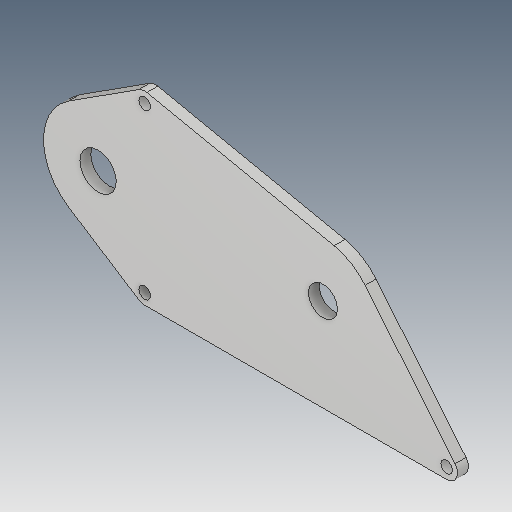
# Autodesk Inventor part: 支え
Saved by Autodesk Inventor 2019.4 (Build 234330000, 330)
## iProperties
Created: 2019-06-12
Part Number: 支え
Material: アルミニウム 2014-T4
Document SubType Name: Modeling
Designer: AzLIer
Density: 2.8 g/cm^3
Appearance: サテン
Mass: 33.3873 g
Surface Area: 90.2364 cm^2
Volume: 11.924 cm^3
Author: AzLIer
Autodesk Inventor part; units mm, degrees
(part 1 of 3)
ref_plane "YZ Plane" through (0, 0, 0) normal (1, 0, 0) x (0, 1, 0)
ref_plane "XZ Plane" through (0, 0, 0) normal (0, 1, 0) x (-1, 0, 0)
ref_plane "XY Plane" through (0, 0, 0) normal (0, 0, 1) x (1, 0, 0)
sketch "スケッチ1" plane through (0, 0, 0) normal (0, 0, 1) x (1, 0, 0)
  circle A0 centre (-1.8122, 42.5) radius 4 construction
  circle A1 centre (60, 42.5) radius 4
  circle A2 centre (0, 0) radius 1.6 construction
  circle A3 centre (120, 0) radius 1.6 construction
  circle A4 centre (-1.8122, 42.5) radius 6 construction
  circle A5 centre (120, 0) radius 1.6 construction
  circle A6 centre (0, 0) radius 1.6 construction
  line L0 (-60, -7.5) -> (5, -7.5) construction
  line L1 (5, -7.5) -> (5, 2.5) construction
  line L2 (5, 2.5) -> (115, 2.5) construction
  line L3 (115, 2.5) -> (115, -7.5) construction
  line L4 (115, -7.5) -> (180, -7.5) construction
  circle A7 centre (60, 42.5) radius 9.5 construction
  circle A8 centre (-1.8122, 42.5) radius 5
  arc A9 (-27.1122, 50.5) -> (-27.1122, 47.5) centre (-27.1122, 49) ccw construction
  line L5 (-27.1122, 50.5) -> (-24.1122, 50.5) construction
  arc A10 (-24.1122, 47.5) -> (-24.1122, 50.5) centre (-24.1122, 49) ccw construction
  line L6 (-24.1122, 47.5) -> (-24.1122, 37.5) construction
  arc A11 (-24.1122, 34.5) -> (-24.1122, 37.5) centre (-24.1122, 36) ccw construction
  line L7 (-24.1122, 34.5) -> (-27.1122, 34.5) construction
  arc A12 (-27.1122, 37.5) -> (-27.1122, 34.5) centre (-27.1122, 36) ccw construction
  line L8 (-27.1122, 37.5) -> (-27.1122, 47.5) construction
  circle A13 centre (-30.1122, 42.5) radius 1.6 construction
  arc A14 (-43.1122, 50.5) -> (-43.1122, 47.5) centre (-43.1122, 49) ccw construction
  line L9 (-43.1122, 50.5) -> (-40.1122, 50.5) construction
  arc A15 (-40.1122, 47.5) -> (-40.1122, 50.5) centre (-40.1122, 49) ccw construction
  line L10 (-40.1122, 47.5) -> (-40.1122, 37.5) construction
  arc A16 (-40.1122, 34.5) -> (-40.1122, 37.5) centre (-40.1122, 36) ccw construction
  line L11 (-40.1122, 34.5) -> (-43.1122, 34.5) construction
  arc A17 (-43.1122, 37.5) -> (-43.1122, 34.5) centre (-43.1122, 36) ccw construction
  line L12 (-43.1122, 37.5) -> (-43.1122, 47.5) construction
  circle A18 centre (-46.1122, 42.5) radius 1.6 construction
  arc A19 (32.7108, 25.7878) -> (79.8762, 17.4214) centre (60, 42.5) ccw construction
  arc A20 (33.6707, 28.6881) -> (32.7108, 25.7878) centre (34.4163, 26.8323) ccw construction
  line L13 (33.6707, 28.6881) -> (46.0418, 33.6587) construction
  arc A21 (48.3419, 33.0614) -> (46.0418, 33.6587) centre (46.7874, 31.8029) ccw construction
  arc A22 (48.3419, 33.0614) -> (71.3533, 32.6969) centre (60, 42.5) ccw construction
  arc A23 (74.6806, 32.2331) -> (71.3533, 32.6969) centre (72.8671, 31.3898) ccw construction
  line L14 (74.6806, 32.2331) -> (80.4475, 19.8322) construction
  arc A24 (79.8762, 17.4214) -> (80.4475, 19.8322) centre (78.634, 18.9888) ccw construction
  arc A25 (45.2156, 45.0341) -> (45.0523, 41.2488) centre (60, 42.5) ccw construction
  arc A26 (43.8049, 39.2261) -> (45.0523, 41.2488) centre (43.0592, 41.0819) ccw construction
  line L15 (43.8049, 39.2261) -> (31.4338, 34.2556) construction
  arc A27 (28.734, 35.6855) -> (31.4338, 34.2556) centre (30.6881, 36.1114) ccw construction
  arc A28 (28.3012, 38.1199) -> (28.734, 35.6855) centre (60, 42.5) ccw construction
  arc A29 (28.2895, 38.5625) -> (28.3012, 38.1199) centre (30.2824, 38.3937) ccw construction
  line L16 (28.2895, 38.5625) -> (29.8074, 56.4773) construction
  arc A30 (33.182, 57.7544) -> (29.8074, 56.4773) centre (31.8002, 56.3085) ccw construction
  line L17 (33.182, 57.7544) -> (44.6261, 46.8179) construction
  arc A31 (45.2156, 45.0341) -> (44.6261, 46.8179) centre (43.2444, 45.372) ccw construction
  arc A32 (37.2786, 112.9254) -> (13.7146, 100.2379) centre (60, 42.5) ccw construction
  arc A33 (39.8605, 111.3796) -> (37.2786, 112.9254) centre (37.8927, 111.022) ccw construction
  line L18 (39.8605, 111.3796) -> (47.3934, 69.926) construction
  arc A34 (44.0438, 68.1225) -> (47.3934, 69.926) centre (45.4256, 69.5684) ccw construction
  line L19 (44.0438, 68.1225) -> (13.5837, 97.2315) construction
  arc A35 (13.7146, 100.2379) -> (13.5837, 97.2315) centre (14.9655, 98.6774) ccw construction
  circle A36 centre (60, 42.5) radius 4 construction
  circle A37 centre (24.575, 76.3537) radius 1.2295 construction
  circle A38 centre (51.2393, 90.7105) radius 1.2295 construction
  circle A39 centre (53.9211, 75.9522) radius 1.2295 construction
  circle A40 centre (35.4194, 65.9903) radius 1.2295 construction
  arc A41 (53.4682, 120.3931) -> (51.2825, 122.0236) centre (51.5004, 120.0355) ccw construction
  arc A42 (51.2825, 122.0236) -> (-1.5901, 93.5555) centre (60, 42.5) ccw construction
  arc A43 (-1.5901, 93.5555) -> (-1.4321, 90.8332) centre (-0.0503, 92.2791) ccw construction
  line L20 (-1.4321, 90.8332) -> (23.8669, 66.6564) construction
  arc A44 (24.4709, 64.9726) -> (23.8669, 66.6564) centre (22.4851, 65.2105) ccw construction
  line L21 (24.4709, 64.9726) -> (22.8037, 51.0517) construction
  arc A45 (20.4778, 49.3186) -> (22.8037, 51.0517) centre (20.8179, 51.2895) ccw construction
  line L22 (20.4778, 49.3186) -> (10.913, 50.9688) construction
  line L23 (10.913, 50.9688) -> (10.8526, 50.6108) construction
  line L24 (10.8526, 50.6108) -> (10.7948, 50.2524) construction
  line L25 (10.7948, 50.2524) -> (10.7396, 49.8936) construction
  line L26 (10.7396, 49.8936) -> (10.687, 49.5343) construction
  line L27 (10.687, 49.5343) -> (10.6371, 49.1747) construction
  line L28 (10.6371, 49.1747) -> (10.5897, 48.8148) construction
  line L29 (10.5897, 48.8148) -> (10.545, 48.4545) construction
  line L30 (10.545, 48.4545) -> (10.5029, 48.0939) construction
  line L31 (10.5029, 48.0939) -> (10.4635, 47.733) construction
  line L32 (10.4635, 47.733) -> (10.4266, 47.3718) construction
  line L33 (10.4266, 47.3718) -> (10.7788, 47.1061) construction
  line L34 (10.7788, 47.1061) -> (11.1328, 46.8484) construction
  line L35 (11.1328, 46.8484) -> (11.4885, 46.5989) construction
  line L36 (11.4885, 46.5989) -> (11.8459, 46.3577) construction
  line L37 (11.8459, 46.3577) -> (12.2048, 46.1249) construction
  line L38 (12.2048, 46.1249) -> (12.5653, 45.9007) construction
  line L39 (12.5653, 45.9007) -> (12.9271, 45.6853) construction
  line L40 (12.9271, 45.6853) -> (13.2903, 45.4788) construction
  line L41 (13.2903, 45.4788) -> (13.6547, 45.2815) construction
  line L42 (13.6547, 45.2815) -> (14.0204, 45.0936) construction
  line L43 (14.0204, 45.0936) -> (14.3872, 44.9154) construction
  line L44 (14.3872, 44.9154) -> (14.755, 44.7473) construction
  line L45 (14.755, 44.7473) -> (15.1238, 44.5897) construction
  line L46 (15.1238, 44.5897) -> (15.4935, 44.4431) construction
  line L47 (15.4935, 44.4431) -> (15.8641, 44.3081) construction
  line L48 (15.8641, 44.3081) -> (16.2354, 44.1857) construction
  line L49 (16.2354, 44.1857) -> (16.6076, 44.077) construction
  line L50 (16.6076, 44.077) -> (16.9805, 43.9839) construction
  line L51 (16.9805, 43.9839) -> (17.3541, 43.9096) construction
  line L52 (17.3541, 43.9096) -> (17.7287, 43.863) construction
  line L53 (17.7287, 43.863) -> (18.0074, 43.843) construction
  line L54 (18.0074, 43.843) -> (18.2771, 43.8116) construction
  line L55 (18.2771, 43.8116) -> (18.5376, 43.771) construction
  line L56 (18.5376, 43.771) -> (18.7888, 43.724) construction
  line L57 (18.7888, 43.724) -> (19.0304, 43.665) construction
  line L58 (19.0304, 43.665) -> (19.2623, 43.5939) construction
  line L59 (19.2623, 43.5939) -> (19.4841, 43.5104) construction
  line L60 (19.4841, 43.5104) -> (19.6958, 43.4209) construction
  line L61 (19.6958, 43.4209) -> (19.897, 43.319) construction
  line L62 (19.897, 43.319) -> (20.0874, 43.2026) construction
  line L63 (20.0874, 43.2026) -> (20.2667, 43.0791) construction
  line L64 (20.2667, 43.0791) -> (20.4346, 42.9419) construction
  line L65 (20.4346, 42.9419) -> (20.5905, 42.7916) construction
  line L66 (20.5905, 42.7916) -> (20.7341, 42.6315) construction
  line L67 (20.7341, 42.6315) -> (20.8645, 42.4541) construction
  line L68 (20.8645, 42.4541) -> (20.9809, 42.2667) construction
  line L69 (20.9809, 42.2667) -> (21.0822, 42.0577) construction
  line L70 (21.0822, 42.0577) -> (21.1667, 41.8325) construction
  line L71 (21.1667, 41.8325) -> (21.2319, 41.5673) construction
  line L72 (21.2319, 41.5673) -> (21.2711, 41.2223) construction
  line L73 (21.2711, 41.2223) -> (21.2729, 41.1669) construction
  line L74 (21.2729, 41.1669) -> (21.2749, 41.1115) construction
  line L75 (21.2749, 41.1115) -> (21.2769, 41.0561) construction
  line L76 (21.2769, 41.0561) -> (21.279, 41.0007) construction
  line L77 (21.279, 41.0007) -> (21.2812, 40.9454) construction
  line L78 (21.2812, 40.9454) -> (21.2835, 40.89) construction
  line L79 (21.2835, 40.89) -> (21.2858, 40.8346) construction
  line L80 (21.2858, 40.8346) -> (21.2882, 40.7793) construction
  line L81 (21.2882, 40.7793) -> (21.2907, 40.7239) construction
  line L82 (21.2907, 40.7239) -> (21.2933, 40.6685) construction
  line L83 (21.2933, 40.6685) -> (21.2819, 40.3215) construction
  line L84 (21.2819, 40.3215) -> (21.2382, 40.0519) construction
  line L85 (21.2382, 40.0519) -> (21.1721, 39.8207) construction
  line L86 (21.1721, 39.8207) -> (21.0878, 39.6042) construction
  line L87 (21.0878, 39.6042) -> (20.9868, 39.4081) construction
  line L88 (20.9868, 39.4081) -> (20.871, 39.2208) construction
  line L89 (20.871, 39.2208) -> (20.7408, 39.0497) construction
  line L90 (20.7408, 39.0497) -> (20.5974, 38.8874) construction
  line L91 (20.5974, 38.8874) -> (20.4411, 38.7371) construction
  line L92 (20.4411, 38.7371) -> (20.2722, 38.5997) construction
  line L93 (20.2722, 38.5997) -> (20.0917, 38.4684) construction
  line L94 (20.0917, 38.4684) -> (19.8994, 38.3507) construction
  line L95 (19.8994, 38.3507) -> (19.6955, 38.2445) construction
  line L96 (19.6955, 38.2445) -> (19.4811, 38.1435) construction
  line L97 (19.4811, 38.1435) -> (19.2557, 38.054) construction
  line L98 (19.2557, 38.054) -> (19.0196, 37.9758) construction
  line L99 (19.0196, 37.9758) -> (18.7729, 37.9089) construction
  line L100 (18.7729, 37.9089) -> (18.5165, 37.8475) construction
  line L101 (18.5165, 37.8475) -> (18.2503, 37.7946) construction
  line L102 (18.2503, 37.7946) -> (17.9741, 37.7523) construction
  line L103 (17.9741, 37.7523) -> (17.6044, 37.6758) construction
  line L104 (17.6044, 37.6758) -> (17.2379, 37.5718) construction
  line L105 (17.2379, 37.5718) -> (16.8737, 37.4491) construction
  line L106 (16.8737, 37.4491) -> (16.5115, 37.3109) construction
  line L107 (16.5115, 37.3109) -> (16.1511, 37.1591) construction
  line L108 (16.1511, 37.1591) -> (15.7926, 36.9949) construction
  line L109 (15.7926, 36.9949) -> (15.4358, 36.8191) construction
  line L110 (15.4358, 36.8191) -> (15.0808, 36.6324) construction
  line L111 (15.0808, 36.6324) -> (14.7277, 36.4354) construction
  line L112 (14.7277, 36.4354) -> (14.3764, 36.2284) construction
  line L113 (14.3764, 36.2284) -> (14.0269, 36.0118) construction
  line L114 (14.0269, 36.0118) -> (13.6795, 35.7859) construction
  line L115 (13.6795, 35.7859) -> (13.334, 35.5509) construction
  line L116 (13.334, 35.5509) -> (12.9906, 35.3072) construction
  line L117 (12.9906, 35.3072) -> (12.6493, 35.0548) construction
  line L118 (12.6493, 35.0548) -> (12.3102, 34.794) construction
  line L119 (12.3102, 34.794) -> (11.9733, 34.5249) construction
  line L120 (11.9733, 34.5249) -> (11.6388, 34.2477) construction
  line L121 (11.6388, 34.2477) -> (11.3066, 33.9624) construction
  line L122 (11.3066, 33.9624) -> (10.9768, 33.6693) construction
  line L123 (10.9768, 33.6693) -> (11.0425, 33.3123) construction
  line L124 (11.0425, 33.3123) -> (11.1108, 32.9557) construction
  line L125 (11.1108, 32.9557) -> (11.1816, 32.5996) construction
  line L126 (11.1816, 32.5996) -> (11.2551, 32.2441) construction
  line L127 (11.2551, 32.2441) -> (11.3311, 31.8891) construction
  line L128 (11.3311, 31.8891) -> (11.4097, 31.5347) construction
  line L129 (11.4097, 31.5347) -> (11.491, 31.1808) construction
  line L130 (11.491, 31.1808) -> (11.5747, 30.8275) construction
  line L131 (11.5747, 30.8275) -> (11.6611, 30.4749) construction
  line L132 (11.6611, 30.4749) -> (11.75, 30.1229) construction
  line L133 (11.75, 30.1229) -> (12.1718, 29.9937) construction
  line L134 (12.1718, 29.9937) -> (12.5926, 29.8726) construction
  line L135 (12.5926, 29.8726) -> (13.0122, 29.7598) construction
  line L136 (13.0122, 29.7598) -> (13.4305, 29.6554) construction
  line L137 (13.4305, 29.6554) -> (13.8474, 29.5594) construction
  line L138 (13.8474, 29.5594) -> (14.2628, 29.472) construction
  line L139 (14.2628, 29.472) -> (14.6765, 29.3933) construction
  line L140 (14.6765, 29.3933) -> (15.0884, 29.3235) construction
  line L141 (15.0884, 29.3235) -> (15.4984, 29.2627) construction
  line L142 (15.4984, 29.2627) -> (15.9062, 29.2112) construction
  line L143 (15.9062, 29.2112) -> (16.3118, 29.1692) construction
  line L144 (16.3118, 29.1692) -> (16.715, 29.1371) construction
  line L145 (16.715, 29.1371) -> (17.1154, 29.1151) construction
  line L146 (17.1154, 29.1151) -> (17.513, 29.1038) construction
  line L147 (17.513, 29.1038) -> (17.9074, 29.1037) construction
  line L148 (17.9074, 29.1037) -> (18.2982, 29.1157) construction
  line L149 (18.2982, 29.1157) -> (18.6851, 29.1409) construction
  line L150 (18.6851, 29.1409) -> (19.0673, 29.1809) construction
  line L151 (19.0673, 29.1809) -> (19.4439, 29.2388) construction
  line L152 (19.4439, 29.2388) -> (19.8118, 29.3232) construction
  line L153 (19.8118, 29.3232) -> (20.0806, 29.3997) construction
  line L154 (20.0806, 29.3997) -> (20.3447, 29.4625) construction
  line L155 (20.3447, 29.4625) -> (20.6033, 29.5133) construction
  line L156 (20.6033, 29.5133) -> (20.8555, 29.5551) construction
  line L157 (20.8555, 29.5551) -> (21.1027, 29.5823) construction
  line L158 (21.1027, 29.5823) -> (21.3449, 29.5948) construction
  line L159 (21.3449, 29.5948) -> (21.5819, 29.5922) construction
  line L160 (21.5819, 29.5922) -> (21.8115, 29.5805) construction
  line L161 (21.8115, 29.5805) -> (22.0354, 29.5535) construction
  line L162 (22.0354, 29.5535) -> (22.2541, 29.5093) construction
  line L163 (22.2541, 29.5093) -> (22.4649, 29.4546) construction
  line L164 (22.4649, 29.4546) -> (22.6695, 29.3831) construction
  line L165 (22.6695, 29.3831) -> (22.8675, 29.2952) construction
  line L166 (22.8675, 29.2952) -> (23.0571, 29.1938) construction
  line L167 (23.0571, 29.1938) -> (23.2403, 29.0717) construction
  line L168 (23.2403, 29.0717) -> (23.4138, 28.9355) construction
  line L169 (23.4138, 28.9355) -> (23.5805, 28.7737) construction
  line L170 (23.5805, 28.7737) -> (23.737, 28.591) construction
  line L171 (23.737, 28.591) -> (23.8889, 28.3641) construction
  line L172 (23.8889, 28.3641) -> (24.0437, 28.0533) construction
  line L173 (24.0437, 28.0533) -> (24.0644, 28.0018) construction
  line L174 (24.0644, 28.0018) -> (24.0852, 27.9505) construction
  line L175 (24.0852, 27.9505) -> (24.106, 27.8991) construction
  line L176 (24.106, 27.8991) -> (24.127, 27.8478) construction
  line L177 (24.127, 27.8478) -> (24.1479, 27.7965) construction
  line L178 (24.1479, 27.7965) -> (24.169, 27.7453) construction
  line L179 (24.169, 27.7453) -> (24.1901, 27.694) construction
  line L180 (24.1901, 27.694) -> (24.2114, 27.6428) construction
  line L181 (24.2114, 27.6428) -> (24.2326, 27.5917) construction
  line L182 (24.2326, 27.5917) -> (24.254, 27.5405) construction
  line L183 (24.254, 27.5405) -> (24.362, 27.2105) construction
  line L184 (24.362, 27.2105) -> (24.4132, 26.9422) construction
  line L185 (24.4132, 26.9422) -> (24.4301, 26.7023) construction
  line L186 (24.4301, 26.7023) -> (24.4249, 26.4701) construction
  line L187 (24.4249, 26.4701) -> (24.397, 26.2513) construction
  line L188 (24.397, 26.2513) -> (24.3523, 26.0357) construction
  line L189 (24.3523, 26.0357) -> (24.2885, 25.8303) construction
  line L190 (24.2885, 25.8303) -> (24.2092, 25.6287) construction
  line L191 (24.2092, 25.6287) -> (24.1137, 25.4341) construction
  line L192 (24.1137, 25.4341) -> (24.0021, 25.2472) construction
  line L193 (24.0021, 25.2472) -> (23.8774, 25.0621) construction
  line L194 (23.8774, 25.0621) -> (23.7369, 24.8857) construction
  line L195 (23.7369, 24.8857) -> (23.5816, 24.7162) construction
  line L196 (23.5816, 24.7162) -> (23.4147, 24.5479) construction
  line L197 (23.4147, 24.5479) -> (23.2335, 24.3868) construction
  line L198 (23.2335, 24.3868) -> (23.0384, 24.2326) construction
  line L199 (23.0384, 24.2326) -> (22.8295, 24.0853) construction
  line L200 (22.8295, 24.0853) -> (22.6096, 23.9399) construction
  line L201 (22.6096, 23.9399) -> (22.3774, 23.7991) construction
  line L202 (22.3774, 23.7991) -> (22.1324, 23.6649) construction
  line L203 (22.1324, 23.6649) -> (21.8111, 23.4666) construction
  line L204 (21.8111, 23.4666) -> (21.5024, 23.2435) construction
  line L205 (21.5024, 23.2435) -> (21.2021, 23.0036) construction
  line L206 (21.2021, 23.0036) -> (20.9089, 22.7499) construction
  line L207 (20.9089, 22.7499) -> (20.6222, 22.484) construction
  line L208 (20.6222, 22.484) -> (20.3415, 22.207) construction
  line L209 (20.3415, 22.207) -> (20.0663, 21.9198) construction
  line L210 (20.0663, 21.9198) -> (19.7966, 21.623) construction
  line L211 (19.7966, 21.623) -> (19.5321, 21.3171) construction
  line L212 (19.5321, 21.3171) -> (19.2728, 21.0024) construction
  line L213 (19.2728, 21.0024) -> (19.0186, 20.6793) construction
  line L214 (19.0186, 20.6793) -> (18.7693, 20.3482) construction
  line L215 (18.7693, 20.3482) -> (18.5251, 20.0093) construction
  line L216 (18.5251, 20.0093) -> (18.2857, 19.6628) construction
  line L217 (18.2857, 19.6628) -> (18.0513, 19.3089) construction
  line L218 (18.0513, 19.3089) -> (17.8219, 18.9478) construction
  line L219 (17.8219, 18.9478) -> (17.5973, 18.5798) construction
  line L220 (17.5973, 18.5798) -> (17.3778, 18.2048) construction
  line L221 (17.3778, 18.2048) -> (17.1632, 17.8232) construction
  line L222 (17.1632, 17.8232) -> (16.9535, 17.435) construction
  line L223 (16.9535, 17.435) -> (17.1374, 17.1219) construction
  line L224 (17.1374, 17.1219) -> (17.3235, 16.8102) construction
  line L225 (17.3235, 16.8102) -> (17.5119, 16.4998) construction
  line L226 (17.5119, 16.4998) -> (17.7025, 16.1908) construction
  line L227 (17.7025, 16.1908) -> (17.8954, 15.8833) construction
  line L228 (17.8954, 15.8833) -> (18.0905, 15.5771) construction
  line L229 (18.0905, 15.5771) -> (18.2878, 15.2724) construction
  line L230 (18.2878, 15.2724) -> (18.4874, 14.9691) construction
  line L231 (18.4874, 14.9691) -> (18.6891, 14.6672) construction
  line L232 (18.6891, 14.6672) -> (18.8931, 14.3669) construction
  line L233 (18.8931, 14.3669) -> (19.3337, 14.3897) construction
  line L234 (19.3337, 14.3897) -> (19.7705, 14.4199) construction
  line L235 (19.7705, 14.4199) -> (20.2033, 14.4574) construction
  line L236 (20.2033, 14.4574) -> (20.6321, 14.5023) construction
  line L237 (20.6321, 14.5023) -> (21.0567, 14.5547) construction
  line L238 (21.0567, 14.5547) -> (21.4769, 14.6146) construction
  line L239 (21.4769, 14.6146) -> (21.8926, 14.6822) construction
  line L240 (21.8926, 14.6822) -> (22.3036, 14.7575) construction
  line L241 (22.3036, 14.7575) -> (22.7096, 14.8406) construction
  line L242 (22.7096, 14.8406) -> (23.1105, 14.9317) construction
  line L243 (23.1105, 14.9317) -> (23.5059, 15.031) construction
  line L244 (23.5059, 15.031) -> (23.8958, 15.1386) construction
  line L245 (23.8958, 15.1386) -> (24.2796, 15.2549) construction
  line L246 (24.2796, 15.2549) -> (24.657, 15.3803) construction
  line L247 (24.657, 15.3803) -> (25.0277, 15.5151) construction
  line L248 (25.0277, 15.5151) -> (25.3908, 15.66) construction
  line L249 (25.3908, 15.66) -> (25.7458, 15.816) construction
  line L250 (25.7458, 15.816) -> (26.0913, 15.9843) construction
  line L251 (26.0913, 15.9843) -> (26.4253, 16.1676) construction
  line L252 (26.4253, 16.1676) -> (26.7422, 16.3727) construction
  line L253 (26.7422, 16.3727) -> (26.9686, 16.5365) construction
  line L254 (26.9686, 16.5365) -> (27.1953, 16.6858) construction
  line L255 (27.1953, 16.6858) -> (27.421, 16.8221) construction
  line L256 (27.421, 16.8221) -> (27.6436, 16.9476) construction
  line L257 (27.6436, 16.9476) -> (27.8666, 17.0577) construction
  line L258 (27.8666, 17.0577) -> (28.0899, 17.1523) construction
  line L259 (28.0899, 17.1523) -> (28.3135, 17.2309) construction
  line L260 (28.3135, 17.2309) -> (28.5333, 17.2984) construction
  line L261 (28.5333, 17.2984) -> (28.7529, 17.3496) construction
  line L262 (28.7529, 17.3496) -> (28.9735, 17.3829) construction
  line L263 (28.9735, 17.3829) -> (29.1903, 17.4036) construction
  line L264 (29.1903, 17.4036) -> (29.4071, 17.4064) construction
  line L265 (29.4071, 17.4064) -> (29.6231, 17.3915) construction
  line L266 (29.6231, 17.3915) -> (29.836, 17.3611) construction
  line L267 (29.836, 17.3611) -> (30.05, 17.309) construction
  line L268 (30.05, 17.309) -> (30.2596, 17.2403) construction
  line L269 (30.2596, 17.2403) -> (30.4716, 17.1453) construction
  line L270 (30.4716, 17.1453) -> (30.6811, 17.0271) construction
  line L271 (30.6811, 17.0271) -> (30.9014, 16.8658) construction
  line L272 (30.9014, 16.8658) -> (31.1532, 16.6267) construction
  line L273 (31.1532, 16.6267) -> (31.1903, 16.5855) construction
  line L274 (31.1903, 16.5855) -> (31.2274, 16.5443) construction
  line L275 (31.2274, 16.5443) -> (31.2645, 16.5032) construction
  line L276 (31.2645, 16.5032) -> (31.3017, 16.4621) construction
  line L277 (31.3017, 16.4621) -> (31.339, 16.4211) construction
  line L278 (31.339, 16.4211) -> (31.3763, 16.3802) construction
  line L279 (31.3763, 16.3802) -> (31.4137, 16.3392) construction
  line L280 (31.4137, 16.3392) -> (31.4511, 16.2984) construction
  line L281 (31.4511, 16.2984) -> (31.4886, 16.2576) construction
  line L282 (31.4886, 16.2576) -> (31.5262, 16.2168) construction
  line L283 (31.5262, 16.2168) -> (31.7405, 15.9436) construction
  line L284 (31.7405, 15.9436) -> (31.8804, 15.7091) construction
  line L285 (31.8804, 15.7091) -> (31.9783, 15.4894) construction
  line L286 (31.9783, 15.4894) -> (32.0529, 15.2694) construction
  line L287 (32.0529, 15.2694) -> (32.1016, 15.0543) construction
  line L288 (32.1016, 15.0543) -> (32.1333, 14.8364) construction
  line L289 (32.1333, 14.8364) -> (32.1435, 14.6216) construction
  line L290 (32.1435, 14.6216) -> (32.138, 14.405) construction
  line L291 (32.138, 14.405) -> (32.1148, 14.1895) construction
  line L292 (32.1148, 14.1895) -> (32.0738, 13.9756) construction
  line L293 (32.0738, 13.9756) -> (32.0199, 13.7591) construction
  line L294 (32.0199, 13.7591) -> (31.9482, 13.5453) construction
  line L295 (31.9482, 13.5453) -> (31.8604, 13.3329) construction
  line L296 (31.8604, 13.3329) -> (31.761, 13.1177) construction
  line L297 (31.761, 13.1177) -> (31.6459, 12.9043) construction
  line L298 (31.6459, 12.9043) -> (31.5153, 12.6926) construction
  line L299 (31.5153, 12.6926) -> (31.3694, 12.4827) construction
  line L300 (31.3694, 12.4827) -> (31.2124, 12.2709) construction
  line L301 (31.2124, 12.2709) -> (31.0424, 12.0593) construction
  line L302 (31.0424, 12.0593) -> (30.8581, 11.8493) construction
  line L303 (30.8581, 11.8493) -> (30.624, 11.5531) construction
  line L304 (30.624, 11.5531) -> (30.4102, 11.2378) construction
  line L305 (30.4102, 11.2378) -> (30.21, 10.9097) construction
  line L306 (30.21, 10.9097) -> (30.0214, 10.571) construction
  line L307 (30.0214, 10.571) -> (29.8429, 10.2231) construction
  line L308 (29.8429, 10.2231) -> (29.6738, 9.8668) construction
  line L309 (29.6738, 9.8668) -> (29.5134, 9.5029) construction
  line L310 (29.5134, 9.5029) -> (29.3615, 9.1317) construction
  line L311 (29.3615, 9.1317) -> (29.2176, 8.7537) construction
  line L312 (29.2176, 8.7537) -> (29.0816, 8.3693) construction
  line L313 (29.0816, 8.3693) -> (28.9532, 7.9788) construction
  line L314 (28.9532, 7.9788) -> (28.8322, 7.5824) construction
  line L315 (28.8322, 7.5824) -> (28.7186, 7.1804) construction
  line L316 (28.7186, 7.1804) -> (28.6122, 6.7729) construction
  line L317 (28.6122, 6.7729) -> (28.513, 6.3602) construction
  line L318 (28.513, 6.3602) -> (28.4208, 5.9424) construction
  line L319 (28.4208, 5.9424) -> (28.3357, 5.5198) construction
  line L320 (28.3357, 5.5198) -> (28.2576, 5.0923) construction
  line L321 (28.2576, 5.0923) -> (28.1865, 4.6603) construction
  line L322 (28.1865, 4.6603) -> (28.1223, 4.2238) construction
  line L323 (28.1223, 4.2238) -> (28.4021, 3.9925) construction
  line L324 (28.4021, 3.9925) -> (28.6836, 3.7632) construction
  line L325 (28.6836, 3.7632) -> (28.9668, 3.536) construction
  line L326 (28.9668, 3.536) -> (29.2516, 3.3109) construction
  line L327 (29.2516, 3.3109) -> (29.538, 3.0878) construction
  line L328 (29.538, 3.0878) -> (29.8261, 2.8668) construction
  line L329 (29.8261, 2.8668) -> (30.1158, 2.648) construction
  line L330 (30.1158, 2.648) -> (30.407, 2.4312) construction
  line L331 (30.407, 2.4312) -> (30.6998, 2.2166) construction
  line L332 (30.6998, 2.2166) -> (30.9942, 2.0041) construction
  line L333 (30.9942, 2.0041) -> (31.4004, 2.1763) construction
  line L334 (31.4004, 2.1763) -> (31.8006, 2.354) construction
  line L335 (31.8006, 2.354) -> (32.1945, 2.5373) construction
  line L336 (32.1945, 2.5373) -> (32.5821, 2.7262) construction
  line L337 (32.5821, 2.7262) -> (32.9631, 2.9206) construction
  line L338 (32.9631, 2.9206) -> (33.3375, 3.1207) construction
  line L339 (33.3375, 3.1207) -> (33.705, 3.3263) construction
  line L340 (33.705, 3.3263) -> (34.0654, 3.5376) construction
  line L341 (34.0654, 3.5376) -> (34.4185, 3.7546) construction
  line L342 (34.4185, 3.7546) -> (34.7641, 3.9773) construction
  line L343 (34.7641, 3.9773) -> (35.1018, 4.2058) construction
  line L344 (35.1018, 4.2058) -> (35.4313, 4.4403) construction
  line L345 (35.4313, 4.4403) -> (35.7522, 4.6809) construction
  line L346 (35.7522, 4.6809) -> (36.064, 4.9278) construction
  line L347 (36.064, 4.9278) -> (36.3661, 5.1812) construction
  line L348 (36.3661, 5.1812) -> (36.6578, 5.4416) construction
  line L349 (36.6578, 5.4416) -> (36.938, 5.7096) construction
  line L350 (36.938, 5.7096) -> (37.2051, 5.986) construction
  line L351 (37.2051, 5.986) -> (37.4563, 6.2724) construction
  line L352 (37.4563, 6.2724) -> (37.684, 6.5735) construction
  line L353 (37.684, 6.5735) -> (37.8407, 6.8049) construction
  line L354 (37.8407, 6.8049) -> (38.0026, 7.0227) construction
  line L355 (38.0026, 7.0227) -> (38.1681, 7.228) construction
  line L356 (38.1681, 7.228) -> (38.3344, 7.4221) construction
  line L357 (38.3344, 7.4221) -> (38.5063, 7.6018) construction
  line L358 (38.5063, 7.6018) -> (38.6838, 7.767) construction
  line L359 (38.6838, 7.767) -> (38.867, 7.9174) construction
  line L360 (38.867, 7.9174) -> (39.0504, 8.056) construction
  line L361 (39.0504, 8.056) -> (39.2393, 8.1793) construction
  line L362 (39.2393, 8.1793) -> (39.4352, 8.286) construction
  line L363 (39.4352, 8.286) -> (39.6318, 8.3795) construction
  line L364 (39.6318, 8.3795) -> (39.8346, 8.4563) construction
  line L365 (39.8346, 8.4563) -> (40.0427, 8.5162) construction
  line L366 (40.0427, 8.5162) -> (40.2532, 8.5604) construction
  line L367 (40.2532, 8.5604) -> (40.472, 8.5847) construction
  line L368 (40.472, 8.5847) -> (40.6925, 8.5918) construction
  line L369 (40.6925, 8.5918) -> (40.9242, 8.5751) construction
  line L370 (40.9242, 8.5751) -> (41.1614, 8.5357) construction
  line L371 (41.1614, 8.5357) -> (41.4237, 8.4595) construction
  line L372 (41.4237, 8.4595) -> (41.7421, 8.3209) construction
  line L373 (41.7421, 8.3209) -> (41.791, 8.2948) construction
  line L374 (41.791, 8.2948) -> (41.8399, 8.2688) construction
  line L375 (41.8399, 8.2688) -> (41.8889, 8.2429) construction
  line L376 (41.8889, 8.2429) -> (41.9379, 8.217) construction
  line L377 (41.9379, 8.217) -> (41.987, 8.1912) construction
  line L378 (41.987, 8.1912) -> (42.036, 8.1655) construction
  line L379 (42.036, 8.1655) -> (42.0852, 8.1398) construction
  line L380 (42.0852, 8.1398) -> (42.1343, 8.1143) construction
  line L381 (42.1343, 8.1143) -> (42.1835, 8.0887) construction
  line L382 (42.1835, 8.0887) -> (42.2327, 8.0633) construction
  line L383 (42.2327, 8.0633) -> (42.5276, 7.8799) construction
  line L384 (42.5276, 7.8799) -> (42.7392, 7.7073) construction
  line L385 (42.7392, 7.7073) -> (42.9064, 7.5344) construction
  line L386 (42.9064, 7.5344) -> (43.0518, 7.3531) construction
  line L387 (43.0518, 7.3531) -> (43.171, 7.1676) construction
  line L388 (43.171, 7.1676) -> (43.2754, 6.9737) construction
  line L389 (43.2754, 6.9737) -> (43.3585, 6.7754) construction
  line L390 (43.3585, 6.7754) -> (43.4273, 6.57) construction
  line L391 (43.4273, 6.57) -> (43.4793, 6.3595) construction
  line L392 (43.4793, 6.3595) -> (43.5139, 6.1445) construction
  line L393 (43.5139, 6.1445) -> (43.5373, 5.9227) construction
  line L394 (43.5373, 5.9227) -> (43.5431, 5.6972) construction
  line L395 (43.5431, 5.6972) -> (43.5331, 5.4675) construction
  line L396 (43.5331, 5.4675) -> (43.5134, 5.2314) construction
  line L397 (43.5134, 5.2314) -> (43.4782, 4.9914) construction
  line L398 (43.4782, 4.9914) -> (43.4278, 4.7479) construction
  line L399 (43.4278, 4.7479) -> (43.3625, 4.5008) construction
  line L400 (43.3625, 4.5008) -> (43.2875, 4.248) construction
  line L401 (43.2875, 4.248) -> (43.2001, 3.991) construction
  line L402 (43.2001, 3.991) -> (43.0987, 3.7307) construction
  line L403 (43.0987, 3.7307) -> (42.9801, 3.3723) construction
  line L404 (42.9801, 3.3723) -> (42.8869, 3.0029) construction
  line L405 (42.8869, 3.0029) -> (42.8111, 2.6261) construction
  line L406 (42.8111, 2.6261) -> (42.7496, 2.2433) construction
  line L407 (42.7496, 2.2433) -> (42.7009, 1.8553) construction
  line L408 (42.7009, 1.8553) -> (42.6639, 1.4627) construction
  line L409 (42.6639, 1.4627) -> (42.6377, 1.0658) construction
  line L410 (42.6377, 1.0658) -> (42.6219, 0.6651) construction
  line L411 (42.6219, 0.6651) -> (42.616, 0.2607) construction
  line L412 (42.616, 0.2607) -> (42.6196, -0.1471) construction
  line L413 (42.6196, -0.1471) -> (42.6325, -0.5579) construction
  line L414 (42.6325, -0.5579) -> (42.6544, -0.9718) construction
  line L415 (42.6544, -0.9718) -> (42.6851, -1.3885) construction
  line L416 (42.6851, -1.3885) -> (42.7245, -1.8077) construction
  line L417 (42.7245, -1.8077) -> (42.7724, -2.2295) construction
  line L418 (42.7724, -2.2295) -> (42.8287, -2.6536) construction
  line L419 (42.8287, -2.6536) -> (42.8933, -3.0799) construction
  line L420 (42.8933, -3.0799) -> (42.9661, -3.5082) construction
  line L421 (42.9661, -3.5082) -> (43.047, -3.9385) construction
  line L422 (43.047, -3.9385) -> (43.136, -4.3706) construction
  line L423 (43.136, -4.3706) -> (43.4781, -4.4923) construction
  line L424 (43.4781, -4.4923) -> (43.821, -4.6115) construction
  line L425 (43.821, -4.6115) -> (44.1648, -4.7281) construction
  line L426 (44.1648, -4.7281) -> (44.5094, -4.8423) construction
  line L427 (44.5094, -4.8423) -> (44.8549, -4.9539) construction
  line L428 (44.8549, -4.9539) -> (45.2011, -5.0631) construction
  line L429 (45.2011, -5.0631) -> (45.5482, -5.1697) construction
  line L430 (45.5482, -5.1697) -> (45.896, -5.2737) construction
  line L431 (45.896, -5.2737) -> (46.2446, -5.3753) construction
  line L432 (46.2446, -5.3753) -> (46.5939, -5.4742) construction
  line L433 (46.5939, -5.4742) -> (46.9167, -5.1735) construction
  line L434 (46.9167, -5.1735) -> (47.2319, -4.8697) construction
  line L435 (47.2319, -4.8697) -> (47.5394, -4.5627) construction
  line L436 (47.5394, -4.5627) -> (47.839, -4.2526) construction
  line L437 (47.839, -4.2526) -> (48.1306, -3.9396) construction
  line L438 (48.1306, -3.9396) -> (48.414, -3.6236) construction
  line L439 (48.414, -3.6236) -> (48.689, -3.3046) construction
  line L440 (48.689, -3.3046) -> (48.9554, -2.9828) construction
  line L441 (48.9554, -2.9828) -> (49.213, -2.6582) construction
  line L442 (49.213, -2.6582) -> (49.4615, -2.3307) construction
  line L443 (49.4615, -2.3307) -> (49.7007, -2.0004) construction
  line L444 (49.7007, -2.0004) -> (49.9301, -1.6674) construction
  line L445 (49.9301, -1.6674) -> (50.1494, -1.3316) construction
  line L446 (50.1494, -1.3316) -> (50.358, -0.9929) construction
  line L447 (50.358, -0.9929) -> (50.5552, -0.6514) construction
  line L448 (50.5552, -0.6514) -> (50.7403, -0.3069) construction
  line L449 (50.7403, -0.3069) -> (50.9119, 0.0407) construction
  line L450 (50.9119, 0.0407) -> (51.0684, 0.3917) construction
  line L451 (51.0684, 0.3917) -> (51.2065, 0.7468) construction
  line L452 (51.2065, 0.7468) -> (51.3174, 1.1076) construction
  line L453 (51.3174, 1.1076) -> (51.3855, 1.3786) construction
  line L454 (51.3855, 1.3786) -> (51.4632, 1.6387) construction
  line L455 (51.4632, 1.6387) -> (51.5485, 1.8882) construction
  line L456 (51.5485, 1.8882) -> (51.6383, 2.1274) construction
  line L457 (51.6383, 2.1274) -> (51.7384, 2.3552) construction
  line L458 (51.7384, 2.3552) -> (51.8487, 2.5711) construction
  line L459 (51.8487, 2.5711) -> (51.9694, 2.7751) construction
  line L460 (51.9694, 2.7751) -> (52.0944, 2.968) construction
  line L461 (52.0944, 2.968) -> (52.2297, 3.1485) construction
  line L462 (52.2297, 3.1485) -> (52.3773, 3.3157) construction
  line L463 (52.3773, 3.3157) -> (52.5301, 3.4709) construction
  line L464 (52.5301, 3.4709) -> (52.6943, 3.6124) construction
  line L465 (52.6943, 3.6124) -> (52.8694, 3.7399) construction
  line L466 (52.8694, 3.7399) -> (53.0521, 3.8534) construction
  line L467 (53.0521, 3.8534) -> (53.2494, 3.951) construction
  line L468 (53.2494, 3.951) -> (53.4541, 4.0332) construction
  line L469 (53.4541, 4.0332) -> (53.6776, 4.0967) construction
  line L470 (53.6776, 4.0967) -> (53.914, 4.1408) construction
  line L471 (53.914, 4.1408) -> (54.1865, 4.1589) construction
  line L472 (54.1865, 4.1589) -> (54.5331, 4.1376) construction
  line L473 (54.5331, 4.1376) -> (54.588, 4.1298) construction
  line L474 (54.588, 4.1298) -> (54.6429, 4.1221) construction
  line L475 (54.6429, 4.1221) -> (54.6978, 4.1145) construction
  line L476 (54.6978, 4.1145) -> (54.7527, 4.1069) construction
  line L477 (54.7527, 4.1069) -> (54.8076, 4.0995) construction
  line L478 (54.8076, 4.0995) -> (54.8625, 4.0921) construction
  line L479 (54.8625, 4.0921) -> (54.9174, 4.0848) construction
  line L480 (54.9174, 4.0848) -> (54.9724, 4.0775) construction
  line L481 (54.9724, 4.0775) -> (55.0273, 4.0704) construction
  line L482 (55.0273, 4.0704) -> (55.0823, 4.0633) construction
  line L483 (55.0823, 4.0633) -> (55.4221, 3.9918) construction
  line L484 (55.4221, 3.9918) -> (55.68, 3.902) construction
  line L485 (55.68, 3.902) -> (55.8962, 3.7967) construction
  line L486 (55.8962, 3.7967) -> (56.0948, 3.6761) construction
  line L487 (56.0948, 3.6761) -> (56.2703, 3.5426) construction
  line L488 (56.2703, 3.5426) -> (56.4347, 3.396) construction
  line L489 (56.4347, 3.396) -> (56.5806, 3.2381) construction
  line L490 (56.5806, 3.2381) -> (56.7156, 3.0687) construction
  line L491 (56.7156, 3.0687) -> (56.8364, 2.8886) construction
  line L492 (56.8364, 2.8886) -> (56.9424, 2.6985) construction
  line L493 (56.9424, 2.6985) -> (57.0403, 2.498) construction
  line L494 (57.0403, 2.498) -> (57.1229, 2.2881) construction
  line L495 (57.1229, 2.2881) -> (57.1921, 2.0689) construction
  line L496 (57.1921, 2.0689) -> (57.2543, 1.8402) construction
  line L497 (57.2543, 1.8402) -> (57.3033, 1.6027) construction
  line L498 (57.3033, 1.6027) -> (57.3393, 1.3566) construction
  line L499 (57.3393, 1.3566) -> (57.3624, 1.102) construction
  line L500 (57.3624, 1.102) -> (57.3783, 0.8389) construction
  line L501 (57.3783, 0.8389) -> (57.3842, 0.5675) construction
  line L502 (57.3842, 0.5675) -> (57.3779, 0.2881) construction
  line L503 (57.3779, 0.2881) -> (57.389, -0.0892) construction
  line L504 (57.389, -0.0892) -> (57.4278, -0.4682) construction
  line L505 (57.4278, -0.4682) -> (57.4854, -0.8482) construction
  line L506 (57.4854, -0.8482) -> (57.5586, -1.2289) construction
  line L507 (57.5586, -1.2289) -> (57.6455, -1.6102) construction
  line L508 (57.6455, -1.6102) -> (57.745, -1.9918) construction
  line L509 (57.745, -1.9918) -> (57.8561, -2.3737) construction
  line L510 (57.8561, -2.3737) -> (57.9783, -2.7557) construction
  line L511 (57.9783, -2.7557) -> (58.111, -3.1377) construction
  line L512 (58.111, -3.1377) -> (58.2539, -3.5196) construction
  line L513 (58.2539, -3.5196) -> (58.4065, -3.9013) construction
  line L514 (58.4065, -3.9013) -> (58.5687, -4.2827) construction
  line L515 (58.5687, -4.2827) -> (58.7401, -4.6637) construction
  line L516 (58.7401, -4.6637) -> (58.9205, -5.0442) construction
  line L517 (58.9205, -5.0442) -> (59.1098, -5.4242) construction
  line L518 (59.1098, -5.4242) -> (59.3077, -5.8034) construction
  line L519 (59.3077, -5.8034) -> (59.5142, -6.1819) construction
  line L520 (59.5142, -6.1819) -> (59.7291, -6.5595) construction
  line L521 (59.7291, -6.5595) -> (59.9523, -6.9362) construction
  line L522 (59.9523, -6.9362) -> (60.1837, -7.3118) construction
  line L523 (60.1837, -7.3118) -> (60.5468, -7.3092) construction
  line L524 (60.5468, -7.3092) -> (60.9098, -7.3039) construction
  line L525 (60.9098, -7.3039) -> (61.2727, -7.2959) construction
  line L526 (61.2727, -7.2959) -> (61.6356, -7.2853) construction
  line L527 (61.6356, -7.2853) -> (61.9985, -7.2721) construction
  line L528 (61.9985, -7.2721) -> (62.3612, -7.2562) construction
  line L529 (62.3612, -7.2562) -> (62.7237, -7.2376) construction
  line L530 (62.7237, -7.2376) -> (63.0862, -7.2165) construction
  line L531 (63.0862, -7.2165) -> (63.4484, -7.1927) construction
  line L532 (63.4484, -7.1927) -> (63.8105, -7.1662) construction
  line L533 (63.8105, -7.1662) -> (64.0111, -6.7732) construction
  line L534 (64.0111, -6.7732) -> (64.2033, -6.3799) construction
  line L535 (64.2033, -6.3799) -> (64.3873, -5.9862) construction
  line L536 (64.3873, -5.9862) -> (64.5628, -5.5924) construction
  line L537 (64.5628, -5.5924) -> (64.7297, -5.1985) construction
  line L538 (64.7297, -5.1985) -> (64.8879, -4.8046) construction
  line L539 (64.8879, -4.8046) -> (65.0372, -4.4109) construction
  line L540 (65.0372, -4.4109) -> (65.1775, -4.0173) construction
  line L541 (65.1775, -4.0173) -> (65.3085, -3.6242) construction
  line L542 (65.3085, -3.6242) -> (65.4301, -3.2314) construction
  line L543 (65.4301, -3.2314) -> (65.5419, -2.8393) construction
  line L544 (65.5419, -2.8393) -> (65.6436, -2.4479) construction
  line L545 (65.6436, -2.4479) -> (65.7347, -2.0573) construction
  line L546 (65.7347, -2.0573) -> (65.8149, -1.6678) construction
  line L547 (65.8149, -1.6678) -> (65.8835, -1.2794) construction
  line L548 (65.8835, -1.2794) -> (65.9395, -0.8924) construction
  line L549 (65.9395, -0.8924) -> (65.9819, -0.507) construction
  line L550 (65.9819, -0.507) -> (66.0089, -0.1236) construction
  line L551 (66.0089, -0.1236) -> (66.0172, 0.2572) construction
  line L552 (66.0172, 0.2572) -> (65.998, 0.6343) construction
  line L553 (65.998, 0.6343) -> (65.9694, 0.9122) construction
  line L554 (65.9694, 0.9122) -> (65.9534, 1.1832) construction
  line L555 (65.9534, 1.1832) -> (65.9482, 1.4468) construction
  line L556 (65.9482, 1.4468) -> (65.9508, 1.7024) construction
  line L557 (65.9508, 1.7024) -> (65.967, 1.9506) construction
  line L558 (65.967, 1.9506) -> (65.9968, 2.1912) construction
  line L559 (65.9968, 2.1912) -> (66.0405, 2.4242) construction
  line L560 (66.0405, 2.4242) -> (66.0919, 2.6482) construction
  line L561 (66.0919, 2.6482) -> (66.1573, 2.864) construction
  line L562 (66.1573, 2.864) -> (66.2388, 3.0717) construction
  line L563 (66.2388, 3.0717) -> (66.3293, 3.2698) construction
  line L564 (66.3293, 3.2698) -> (66.4353, 3.4589) construction
  line L565 (66.4353, 3.4589) -> (66.5562, 3.6386) construction
  line L566 (66.5562, 3.6386) -> (66.689, 3.8078) construction
  line L567 (66.689, 3.8078) -> (66.8411, 3.967) construction
  line L568 (66.8411, 3.967) -> (67.0053, 4.1142) construction
  line L569 (67.0053, 4.1142) -> (67.1936, 4.2503) construction
  line L570 (67.1936, 4.2503) -> (67.4007, 4.3726) construction
  line L571 (67.4007, 4.3726) -> (67.6505, 4.4828) construction
  line L572 (67.6505, 4.4828) -> (67.9835, 4.5813) construction
  line L573 (67.9835, 4.5813) -> (68.0378, 4.5928) construction
  line L574 (68.0378, 4.5928) -> (68.092, 4.6043) construction
  line L575 (68.092, 4.6043) -> (68.1461, 4.6159) construction
  line L576 (68.1461, 4.6159) -> (68.2003, 4.6276) construction
  line L577 (68.2003, 4.6276) -> (68.2545, 4.6394) construction
  line L578 (68.2545, 4.6394) -> (68.3086, 4.6512) construction
  line L579 (68.3086, 4.6512) -> (68.3627, 4.6632) construction
  line L580 (68.3627, 4.6632) -> (68.4168, 4.6752) construction
  line L581 (68.4168, 4.6752) -> (68.4709, 4.6872) construction
  line L582 (68.4709, 4.6872) -> (68.525, 4.6994) construction
  line L583 (68.525, 4.6994) -> (68.8688, 4.7484) construction
  line L584 (68.8688, 4.7484) -> (69.1418, 4.7522) construction
  line L585 (69.1418, 4.7522) -> (69.381, 4.7272) construction
  line L586 (69.381, 4.7272) -> (69.6089, 4.6818) construction
  line L587 (69.6089, 4.6818) -> (69.8195, 4.6164) construction
  line L588 (69.8195, 4.6164) -> (70.0241, 4.5349) construction
  line L589 (70.0241, 4.5349) -> (70.2152, 4.4364) construction
  line L590 (70.2152, 4.4364) -> (70.4, 4.3233) construction
  line L591 (70.4, 4.3233) -> (70.575, 4.1955) construction
  line L592 (70.575, 4.1955) -> (70.7398, 4.053) construction
  line L593 (70.7398, 4.053) -> (70.9003, 3.8981) construction
  line L594 (70.9003, 3.8981) -> (71.0497, 3.7291) construction
  line L595 (71.0497, 3.7291) -> (71.1897, 3.5468) construction
  line L596 (71.1897, 3.5468) -> (71.3264, 3.3532) construction
  line L597 (71.3264, 3.3532) -> (71.4536, 3.1468) construction
  line L598 (71.4536, 3.1468) -> (71.5716, 2.9278) construction
  line L599 (71.5716, 2.9278) -> (71.6804, 2.6965) construction
  line L600 (71.6804, 2.6965) -> (71.7854, 2.4547) construction
  line L601 (71.7854, 2.4547) -> (71.8837, 2.2016) construction
  line L602 (71.8837, 2.2016) -> (71.9733, 1.937) construction
  line L603 (71.9733, 1.937) -> (72.1128, 1.5862) construction
  line L604 (72.1128, 1.5862) -> (72.2789, 1.2434) construction
  line L605 (72.2789, 1.2434) -> (72.463, 0.906) construction
  line L606 (72.463, 0.906) -> (72.662, 0.5733) construction
  line L607 (72.662, 0.5733) -> (72.874, 0.2447) construction
  line L608 (72.874, 0.2447) -> (73.098, -0.0799) construction
  line L609 (73.098, -0.0799) -> (73.3331, -0.4007) construction
  line L610 (73.3331, -0.4007) -> (73.5786, -0.7179) construction
  line L611 (73.5786, -0.7179) -> (73.834, -1.0314) construction
  line L612 (73.834, -1.0314) -> (74.0988, -1.3415) construction
  line L613 (74.0988, -1.3415) -> (74.3728, -1.6479) construction
  line L614 (74.3728, -1.6479) -> (74.6556, -1.9509) construction
  line L615 (74.6556, -1.9509) -> (74.947, -2.2503) construction
  line L616 (74.947, -2.2503) -> (75.2467, -2.5462) construction
  line L617 (75.2467, -2.5462) -> (75.5545, -2.8385) construction
  line L618 (75.5545, -2.8385) -> (75.8702, -3.1271) construction
  line L619 (75.8702, -3.1271) -> (76.1937, -3.4122) construction
  line L620 (76.1937, -3.4122) -> (76.5248, -3.6935) construction
  line L621 (76.5248, -3.6935) -> (76.8634, -3.9711) construction
  line L622 (76.8634, -3.9711) -> (77.2093, -4.245) construction
  line L623 (77.2093, -4.245) -> (77.5495, -4.1183) construction
  line L624 (77.5495, -4.1183) -> (77.8888, -3.9891) construction
  line L625 (77.8888, -3.9891) -> (78.2272, -3.8575) construction
  line L626 (78.2272, -3.8575) -> (78.5646, -3.7235) construction
  line L627 (78.5646, -3.7235) -> (78.901, -3.5869) construction
  line L628 (78.901, -3.5869) -> (79.2364, -3.4479) construction
  line L629 (79.2364, -3.4479) -> (79.5708, -3.3065) construction
  line L630 (79.5708, -3.3065) -> (79.9041, -3.1627) construction
  line L631 (79.9041, -3.1627) -> (80.2364, -3.0164) construction
  line L632 (80.2364, -3.0164) -> (80.5676, -2.8677) construction
  line L633 (80.5676, -2.8677) -> (80.6216, -2.4298) construction
  line L634 (80.6216, -2.4298) -> (80.6678, -1.9944) construction
  line L635 (80.6678, -1.9944) -> (80.706, -1.5616) construction
  line L636 (80.706, -1.5616) -> (80.7362, -1.1315) construction
  line L637 (80.7362, -1.1315) -> (80.7583, -0.7043) construction
  line L638 (80.7583, -0.7043) -> (80.7723, -0.28) construction
  line L639 (80.7723, -0.28) -> (80.7779, 0.141) construction
  line L640 (80.7779, 0.141) -> (80.7751, 0.5588) construction
  line L641 (80.7751, 0.5588) -> (80.7638, 0.9731) construction
  line L642 (80.7638, 0.9731) -> (80.7437, 1.3837) construction
  line L643 (80.7437, 1.3837) -> (80.7146, 1.7904) construction
  line L644 (80.7146, 1.7904) -> (80.6763, 2.193) construction
  line L645 (80.6763, 2.193) -> (80.6284, 2.5912) construction
  line L646 (80.6284, 2.5912) -> (80.5705, 2.9847) construction
  line L647 (80.5705, 2.9847) -> (80.5021, 3.3731) construction
  line L648 (80.5021, 3.3731) -> (80.4224, 3.7559) construction
  line L649 (80.4224, 3.7559) -> (80.3305, 4.1326) construction
  line L650 (80.3305, 4.1326) -> (80.2247, 4.502) construction
  line L651 (80.2247, 4.502) -> (80.1022, 4.8628) construction
  line L652 (80.1022, 4.8628) -> (79.9552, 5.2105) construction
  line L653 (79.9552, 5.2105) -> (79.8332, 5.4619) construction
  line L654 (79.8332, 5.4619) -> (79.7256, 5.7111) construction
  line L655 (79.7256, 5.7111) -> (79.6305, 5.957) construction
  line L656 (79.6305, 5.957) -> (79.5456, 6.1981) construction
  line L657 (79.5456, 6.1981) -> (79.4759, 6.4368) construction
  line L658 (79.4759, 6.4368) -> (79.4215, 6.6731) construction
  line L659 (79.4215, 6.6731) -> (79.3829, 6.907) construction
  line L660 (79.3829, 6.907) -> (79.3546, 7.1351) construction
  line L661 (79.3546, 7.1351) -> (79.3423, 7.3603) construction
  line L662 (79.3423, 7.3603) -> (79.3478, 7.5833) construction
  line L663 (79.3478, 7.5833) -> (79.3651, 7.8004) construction
  line L664 (79.3651, 7.8004) -> (79.4, 8.0144) construction
  line L665 (79.4, 8.0144) -> (79.4522, 8.2246) construction
  line L666 (79.4522, 8.2246) -> (79.5191, 8.429) construction
  line L667 (79.5191, 8.429) -> (79.6076, 8.6306) construction
  line L668 (79.6076, 8.6306) -> (79.7116, 8.8251) construction
  line L669 (79.7116, 8.8251) -> (79.8419, 9.0174) construction
  line L670 (79.8419, 9.0174) -> (79.9947, 9.2032) construction
  line L671 (79.9947, 9.2032) -> (80.1918, 9.3922) construction
  line L672 (80.1918, 9.3922) -> (80.471, 9.5986) construction
  line L673 (80.471, 9.5986) -> (80.518, 9.628) construction
  line L674 (80.518, 9.628) -> (80.565, 9.6573) construction
  line L675 (80.565, 9.6573) -> (80.612, 9.6868) construction
  line L676 (80.612, 9.6868) -> (80.6589, 9.7163) construction
  line L677 (80.6589, 9.7163) -> (80.7058, 9.7459) construction
  line L678 (80.7058, 9.7459) -> (80.7526, 9.7755) construction
  line L679 (80.7526, 9.7755) -> (80.7994, 9.8052) construction
  line L680 (80.7994, 9.8052) -> (80.8461, 9.835) construction
  line L681 (80.8461, 9.835) -> (80.8928, 9.8648) construction
  line L682 (80.8928, 9.8648) -> (80.9394, 9.8948) construction
  line L683 (80.9394, 9.8948) -> (81.2457, 10.0584) construction
  line L684 (81.2457, 10.0584) -> (81.501, 10.1554) construction
  line L685 (81.501, 10.1554) -> (81.7344, 10.2137) construction
  line L686 (81.7344, 10.2137) -> (81.964, 10.249) construction
  line L687 (81.964, 10.249) -> (82.1843, 10.2595) construction
  line L688 (82.1843, 10.2595) -> (82.4044, 10.2529) construction
  line L689 (82.4044, 10.2529) -> (82.6177, 10.2257) construction
  line L690 (82.6177, 10.2257) -> (82.83, 10.1827) construction
  line L691 (82.83, 10.1827) -> (83.0382, 10.1224) construction
  line L692 (83.0382, 10.1224) -> (83.2417, 10.0449) construction
  line L693 (83.2417, 10.0449) -> (83.4456, 9.9542) construction
  line L694 (83.4456, 9.9542) -> (83.6437, 9.8465) construction
  line L695 (83.6437, 9.8465) -> (83.8376, 9.7231) construction
  line L696 (83.8376, 9.7231) -> (84.0323, 9.5879) construction
  line L697 (84.0323, 9.5879) -> (84.2225, 9.4374) construction
  line L698 (84.2225, 9.4374) -> (84.4082, 9.272) construction
  line L699 (84.4082, 9.272) -> (84.5896, 9.0919) construction
  line L700 (84.5896, 9.0919) -> (84.771, 8.9005) construction
  line L701 (84.771, 8.9005) -> (84.9499, 8.6964) construction
  line L702 (84.9499, 8.6964) -> (85.1246, 8.4784) construction
  line L703 (85.1246, 8.4784) -> (85.3756, 8.1964) construction
  line L704 (85.3756, 8.1964) -> (85.649, 7.9311) construction
  line L705 (85.649, 7.9311) -> (85.9374, 7.677) construction
  line L706 (85.9374, 7.677) -> (86.2382, 7.4324) construction
  line L707 (86.2382, 7.4324) -> (86.5498, 7.1962) construction
  line L708 (86.5498, 7.1962) -> (86.8713, 6.9678) construction